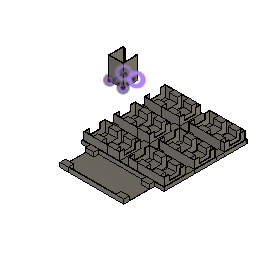
ScotlandYardInsert (Autodesk Fusion 360 design; units mm, degrees)
Autodesk Fusion 360 part; units mm, degrees
sketch "Sketch1" plane through (0, 0, 0) normal (0, 0, 1) x (1, 0, 0)
  line L0 (0, 0) -> (149.4, 0)
  line L1 (149.4, 0) -> (149.4, -151.8)
  line L2 (149.4, -151.8) -> (0, -151.8)
  line L3 (0, -151.8) -> (0, 0)
  line L4 (1.2, -1.2) -> (67.2, -1.2)
  line L5 (67.2, -1.2) -> (67.2, -41)
  line L6 (67.2, -41) -> (1.2, -41)
  line L7 (1.2, -41) -> (1.2, -1.2)
  line L8 (82.2, -1.2) -> (148.2, -1.2)
  line L9 (148.2, -41) -> (82.2, -41)
  line L10 (82.2, -41) -> (82.2, -1.2)
  line L11 (148.2, -1.2) -> (148.2, -41)
  line L12 (1.2, -56) -> (67.2, -56)
  line L13 (67.2, -95.8) -> (1.2, -95.8)
  line L14 (1.2, -95.8) -> (1.2, -56)
  line L15 (67.2, -56) -> (67.2, -95.8)
  line L16 (1.2, -110.8) -> (67.2, -110.8)
  line L17 (67.2, -150.6) -> (1.2, -150.6)
  line L18 (1.2, -150.6) -> (1.2, -110.8)
  line L19 (67.2, -110.8) -> (67.2, -150.6)
  line L20 (82.2, -56) -> (148.2, -56)
  line L21 (148.2, -95.8) -> (82.2, -95.8)
  line L22 (82.2, -95.8) -> (82.2, -56)
  line L23 (148.2, -56) -> (148.2, -95.8)
  line L24 (82.2, -110.8) -> (148.2, -110.8)
  line L25 (148.2, -150.6) -> (82.2, -150.6)
  line L26 (82.2, -150.6) -> (82.2, -110.8)
  line L27 (148.2, -110.8) -> (148.2, -150.6)
  line L28 (16.7, -151.8) -> (132.7, -151.8)
  line L29 (132.7, -151.8) -> (132.7, -208.4)
  line L30 (132.7, -208.4) -> (16.7, -208.4)
  line L31 (16.7, -208.4) -> (16.7, -151.8)
  line L32 (31.7, -153) -> (117.7, -153)
  line L33 (117.7, -153) -> (117.7, -207.2)
  line L34 (117.7, -207.2) -> (31.7, -207.2)
  line L35 (31.7, -207.2) -> (31.7, -153)
  dimension "d1" = 66
  dimension "d2" = 39.8
  dimension "d3" = 66
  dimension "d13" = 1.2
  dimension "d14" = 1.2
  dimension "d15" = 15
  dimension "d16" = 15
  dimension "d17" = 39.8
  dimension "d18" = 39.8
  dimension "d19" = 15
  dimension "d20" = 1.2
  dimension "d21" = 1.2
  dimension "d28" = 1.2
  dimension "d29" = 15
  dimension "d30" = 15
  dimension "d31" = 1.2
  dimension "d32" = 86
  dimension "d33" = 54.2
  constraint horizontal L0
  constraint vertical L1
  constraint horizontal L2
  constraint vertical L3
  constraint coincident L0.start L3.end
  constraint horizontal L4
  constraint vertical L5
  constraint horizontal L6
  constraint vertical L7
  constraint horizontal L8
  constraint vertical L11
  constraint horizontal L9
  constraint vertical L10
  constraint horizontal L12
  constraint vertical L15
  constraint horizontal L13
  constraint vertical L14
  constraint horizontal L16
  constraint vertical L19
  constraint horizontal L17
  constraint vertical L18
  constraint horizontal L20
  constraint vertical L23
  constraint horizontal L21
  constraint vertical L22
  constraint horizontal L24
  constraint vertical L27
  constraint horizontal L25
  constraint vertical L26
  constraint coincident L4.end L8
  constraint coincident L5.end L9
  constraint coincident L6.end L14
  constraint coincident L5.end L15
  constraint coincident L9.end L22
  constraint coincident L12.end L20
  constraint coincident L13.start L21
  constraint coincident L9.start L23
  constraint coincident L13.end L18
  constraint coincident L13.start L19
  constraint coincident L16.end L24
  constraint coincident L17.start L25
  constraint coincident L21.end L26
  constraint coincident L21.start L27
  constraint horizontal L28
  constraint vertical L29
  constraint horizontal L30
  constraint vertical L31
  constraint coincident L2 L28.start
  constraint horizontal L32
  constraint vertical L33
  constraint horizontal L34
  constraint vertical L35
  constraint midpoint L2 L28
  measures "d1" distance of L5 L7
  measures "d2" distance of L4 L6
  measures "d3" distance of L10 L11
  measures "d13" distance of L0 L4
  measures "d14" distance of L3 L7
  measures "d15" distance of L5 L10
  measures "d16" distance of L6 L12
  measures "d17" distance of L12 L13
  measures "d18" distance of L16 L17
  measures "d19" distance of L13 L16
  measures "d20" distance of L2 L17
  measures "d21" distance of L1 L27
  measures "d28" distance of L2 L32
  measures "d29" distance of L31 L35
  measures "d30" distance of L29 L33
  measures "d31" distance of L30 L34
  measures "d32" distance of L33 L35
  measures "d33" distance of L32 L34
extrude "Extrude1" add sketch "Sketch1" along normal blind 0.6 contours L4 L5 L6 L7 | L8 L9 L10 L11 | L12 L13 L14 L15 | L16 L17 L18 L19 | L20 L21 L22 L23 | L24 L25 L26 L27 makes body 1 at (23.2, -69.2667, 0) makes body 2 at (23.2, -14.4667, 0) makes body 3 at (45.2, -137.3333, 0) makes body 4 at (104.2, -69.2667, 0) makes body 5 at (126.2, -14.4667, 0) makes body 6 at (104.2, -124.0667, 0)
extrude "Extrude2" add sketch "Sketch1" along normal blind 6.6 contours L0 L1 L2 L3 L28 bodies 1 2 3 4 5 6
extrude "Extrude3" add sketch "Sketch1" along normal blind 0.6 separate body contours L32 L33 L34 L35 makes body 7
extrude "Extrude4" add sketch "Sketch1" along normal blind 8 contours L2 L28 L29 L30 L31 bodies 1 7
sketch "Sketch2" plane through (132.7, 0, 0) normal (1, 0, 0) x (0, 1, 0)
  line L0 (-208.4, 0) -> (-151.8, 0)
  line L1 (-151.8, 0) -> (-151.8, 6.6)
  line L2 (-151.8, 6.6) -> (-151.8, 8)
  line L3 (-151.8, 8) -> (-208.4, 8)
  line L4 (-208.4, 8) -> (-208.4, 0)
  line L5 (-198.4, 8) -> (-161.8, 8)
  line L6 (-161.8, 8) -> (-161.8, 0.6)
  line L7 (-161.8, 0.6) -> (-198.4, 0.6)
  line L8 (-198.4, 0.6) -> (-198.4, 8)
  line L9 (-151.8, 0) -> (-208.4, 0)
  dimension "d40" = 0.6
  dimension "d41" = 10
  constraint horizontal L5
  constraint vertical L6
  constraint horizontal L7
  constraint vertical L8
  constraint coincident L3 L5.start
  constraint midpoint L3 L5
  measures "d40" distance of L7 L9
  measures "d41" distance of L4 L8
extrude "Extrude5" cut sketch "Sketch2" against normal blind 116 contours L3 L5 L6 L7 L8 bodies 1
sketch "Sketch4" plane through (0, 0, 0) normal (0, 1, 0) x (-1, 0, 0)
  line L0 (-149.4, 0) -> (0, 0)
  line L1 (0, 0) -> (0, 6.6)
  line L2 (0, 6.6) -> (-149.4, 6.6)
  line L3 (-149.4, 6.6) -> (-149.4, 0)
  line L4 (-57.2, 6.6) -> (-11.2, 6.6)
  line L5 (-11.2, 6.6) -> (-11.2, 2)
  line L6 (-11.2, 2) -> (-57.2, 2)
  line L7 (-57.2, 2) -> (-57.2, 6.6)
  line L8 (-67.2, 6.6) -> (-1.2, 6.6)
  line L9 (0, 0) -> (-149.4, 0)
  line L10 (-74.7, 0) -> (-74.7, 6.6)
  line L11 (-92.2, 2) -> (-92.2, 6.6)
  line L12 (-138.2, 2) -> (-92.2, 2)
  line L13 (-92.2, 6.6) -> (-138.2, 6.6)
  line L14 (-138.2, 6.6) -> (-138.2, 2)
  dimension "d50" = 2
  dimension "d51" = 10
  constraint horizontal L4
  constraint vertical L5
  constraint horizontal L6
  constraint vertical L7
  constraint coincident L2 L4.start
  constraint midpoint L4 L8
  constraint coincident L9 L10.start
  constraint coincident L2 L10.end
  constraint perpendicular L2 L10
  constraint midpoint L2 L10.end
  constraint symmetric L4.start L10 L11.end
  constraint symmetric L4.end L10 L13.end
  constraint symmetric L5.end L10 L12.start
  constraint symmetric L6.end L10 L11.start
  measures "d50" distance of L6 L9
  measures "d51" distance of L7 L8.start
extrude "Extrude8" cut sketch "Sketch4" against normal blind 111 contours L2 L11 L12 L13 L14 | L2 L4 L5 L6 L7 L8 bodies 1
sketch "Sketch1 (2)" plane through (0, 0, 0) normal (0, 0, 1) x (1, 0, 0) in component "Krabicka"
  line L0 (66.6, -40.4) -> (1.8, -40.4)
  line L1 (1.8, -40.4) -> (1.8, -1.8)
  line L2 (1.8, -1.8) -> (66.6, -1.8)
  line L3 (66.6, -1.8) -> (66.6, -40.4)
  line L4 (65.4, -39.2) -> (59.2, -39.2)
  line L5 (59.2, -39.2) -> (59.2, -3)
  line L6 (59.2, -3) -> (65.4, -3)
  line L7 (65.4, -3) -> (65.4, -39.2)
  line L8 (44.2, -39.2) -> (33, -39.2)
  line L9 (33, -39.2) -> (33, -3)
  line L10 (33, -3) -> (44.2, -3)
  line L11 (44.2, -3) -> (44.2, -39.2)
  line L12 (18, -39.2) -> (3, -39.2)
  line L13 (3, -39.2) -> (3, -3)
  line L14 (3, -3) -> (18, -3)
  line L15 (18, -3) -> (18, -39.2)
  line L16 (67.2, -1.2) -> (67.2, -41)
  line L17 (67.2, -41) -> (57.2, -41)
  line L18 (57.2, -1.2) -> (67.2, -1.2)
  dimension "d56" = 6.2
  dimension "d57" = 1.2
  dimension "d58" = 15
  dimension "d59" = 11.2
  dimension "d60" = 15
  dimension "d61" = 15
  dimension "d62" = 1.2
  dimension "d63" = 1.2
  dimension "d74" = 1.2
  dimension "d76" = 0.6
  dimension "d77" = 0.6
  dimension "d78" = 0.6
  constraint horizontal L0
  constraint vertical L1
  constraint horizontal L2
  constraint vertical L3
  constraint horizontal L4
  constraint vertical L5
  constraint horizontal L6
  constraint vertical L7
  constraint horizontal L8
  constraint vertical L9
  constraint horizontal L10
  constraint vertical L11
  constraint horizontal L12
  constraint vertical L13
  constraint horizontal L14
  constraint vertical L15
  constraint coincident L9.end L14
  constraint coincident L5.end L10
  constraint coincident L4 L8.start
  constraint coincident L8 L12.start
  measures "d56" distance of L5 L7
  measures "d57" distance of L3 L7
  measures "d58" distance of L5 L11
  measures "d59" distance of L9 L11
  measures "d60" distance of L9 L15
  measures "d61" distance of L13 L15
  measures "d62" distance of L2 L6
  measures "d63" distance of L0 L4
  measures "d74" distance of L1 L13
  measures "d76" distance of L0 L17
  measures "d77" distance of L3 L16
  measures "d78" distance of L2 L18
extrude "Extrude1'" add sketch "Sketch1 (2)" along normal blind 0.6 separate body contours L4 L5 L6 L7 | L8 L9 L10 L11 | L12 L13 L14 L15 makes body 8 at (8, -27.1333, 0) makes body 9 at (40.4667, -27.1333, 0) makes body 10 at (61.2667, -27.1333, 0) in component "Krabicka"
extrude "Extrude2'" add sketch "Sketch1 (2)" along normal blind 20 bodies 8 9 10 in component "Krabicka"
sketch "Sketch2 (2)" plane through (66.6, 0, 0) normal (1, 0, 0) x (0, 1, 0) in component "Krabicka"
  line L0 (-40.4, 0) -> (-1.8, 0)
  line L1 (-1.8, 0) -> (-1.8, 20)
  line L2 (-1.8, 20) -> (-40.4, 20)
  line L3 (-40.4, 20) -> (-40.4, 0)
  line L4 (-31.1, 20) -> (-11.1, 20)
  line L5 (-11.1, 20) -> (-11.1, 10)
  line L6 (-11.1, 10) -> (-31.1, 10)
  line L7 (-31.1, 10) -> (-31.1, 20)
  dimension "d70" = 10
  dimension "d71" = 20
  constraint horizontal L4
  constraint vertical L5
  constraint horizontal L6
  constraint vertical L7
  constraint coincident L2 L4.start
  constraint midpoint L2 L4
  measures "d70" distance of L4 L6
  measures "d71" distance of L5 L7
extrude "Extrude3'" cut sketch "Sketch2 (2)" against normal blind 64.8 contours L2 L4 L5 L6 L7 bodies 8 in component "Krabicka"
pattern_linear "00000000-0000-0000-0000-000000000000" [suppressed]
pattern_linear "R-Pattern1" count 3 spacing 54.8 along (0, -1, 0) count 2 spacing 81 along (1, 0, 0) of bodies 8 makes body 11 at (23.4, -82.3333, 0) makes body 12 at (23.4, -137.1333, 0) makes body 13 at (104.4, -27.5333, 0) makes body 14 at (104.4, -82.3333, 0) makes body 15 at (104.4, -137.1333, 0) in component "Krabicka"
sketch "Sketch1 (3)" plane through (0, 0, 0) normal (0, 0, 1) x (1, 0, 0) in component "VytahovaciStojan"
  line L0 (-50, 0) -> (-76.8, 0)
  line L1 (-76.8, 0) -> (-76.8, -26.8)
  line L2 (-76.8, -26.8) -> (-50, -26.8)
  line L3 (-50, -26.8) -> (-50, 0)
  line L4 (-51.2, -25.6) -> (-75.6, -25.6)
  line L5 (-75.6, -25.6) -> (-75.6, -1.2)
  line L6 (-75.6, -1.2) -> (-51.2, -1.2)
  line L7 (-51.2, -1.2) -> (-51.2, -25.6)
  dimension "d87" = 26.8
  dimension "d88" = 26.8
  dimension "d90" = 1.2
  dimension "d91" = 1.2
  dimension "d93" = 1.2
  dimension "d94" = 1.2
  dimension "d96" = 50
  constraint horizontal L0
  constraint vertical L1
  constraint horizontal L2
  constraint vertical L3
  constraint horizontal L4
  constraint vertical L5
  constraint horizontal L6
  constraint vertical L7
  constraint coincident origin L0
  measures "d87" distance of L0.start L0.end
  measures "d88" distance of L0 L2
  measures "d90" distance of L3 L7
  measures "d91" distance of L0 L6
  measures "d93" distance of L2 L4
  measures "d94" distance of L1 L5
  measures "d96" distance of origin L3
extrude "Extrude1''" add sketch "Sketch1 (3)" along normal blind 0.6 separate body contours L4 L5 L6 L7 makes body 16 in component "VytahovaciStojan"
extrude "Extrude2''" add sketch "Sketch1 (3)" along normal blind 39.6 bodies 16 in component "VytahovaciStojan"
sketch "Sketch2 (3)" plane through (0, 0, 0) normal (0, 1, 0) x (-1, 0, 0) in component "VytahovaciStojan"
  line L0 (50, 0) -> (76.8, 0)
  line L1 (76.8, 0) -> (76.8, 39.6)
  line L2 (76.8, 39.6) -> (50, 39.6)
  line L3 (50, 39.6) -> (50, 0)
  line L4 (52, 1.8) -> (54, 5.8)
  line L5 (54, 11.6641) -> (54, 39.6)
  line L6 (54, 5.8) -> (54, 7)
  line L7 (54, 7) -> (52, 7)
  line L8 (52, 1.8) -> (52, 0.6)
  line L9 (52, 0.6) -> (54, 0.6)
  line L10 (54, 0.6) -> (54, 0)
  line L11 (52, 7) -> (52, 8.2)
  line L12 (52, 8.2) -> (54, 11.6641)
  line L13 (50, 0) -> (76.8, 0)
  line L14 (63.4, 0) -> (63.4, 39.6)
  line L15 (72.8, 11.6641) -> (72.8, 39.6)
  line L16 (74.8, 8.2) -> (72.8, 11.6641)
  line L17 (74.8, 7) -> (74.8, 8.2)
  line L18 (72.8, 7) -> (74.8, 7)
  line L19 (72.8, 5.8) -> (72.8, 7)
  line L20 (74.8, 1.8) -> (72.8, 5.8)
  line L21 (74.8, 1.8) -> (74.8, 0.6)
  line L22 (74.8, 0.6) -> (72.8, 0.6)
  line L23 (72.8, 0.6) -> (72.8, 0)
  dimension "d101" = 4
  dimension "d110" = 0.6
  dimension "d111" = 1.2
  dimension "d112" = 1.2
  dimension "d113" = 2
  dimension "d114" = 1.2
  dimension "d117" = 30
  dimension "d120" = 4
  dimension "d121" = 3.4641
  constraint coincident L2 L5.end
  constraint perpendicular L2 L5
  constraint vertical L6
  constraint perpendicular L6 L7
  constraint parallel L3 L8
  constraint perpendicular L8 L9
  constraint coincident L0 L10.end
  constraint perpendicular L0 L10
  constraint perpendicular L7 L11
  constraint coincident L5.start L12.end
  constraint coincident L7.end L8
  constraint midpoint L0 L14.start
  constraint midpoint L2 L14.end
  constraint coincident L4.end L10
  constraint symmetric L4.start L14 L20.start
  constraint symmetric L4.end L14 L19.start
  constraint symmetric L5.start L14 L15.start
  constraint symmetric L5.end L14 L15.end
  constraint symmetric L6.end L14 L18.start
  constraint symmetric L7.end L14 L17.start
  constraint symmetric L8.end L14 L21.end
  constraint symmetric L9.end L14 L22.end
  constraint symmetric L10.end L14 L23.end
  constraint symmetric L11.end L14 L16.start
  measures "d101" distance of L3 L5
  measures "d110" distance of L9 L13
  measures "d111" distance of L4.end L6.end
  measures "d112" distance of L4.start L8.end
  measures "d113" distance of L6.end L7.end
  measures "d114" distance of L7.end L11.end
  measures "d117" angle of L5 L12
  measures "d120" vertical distance of L4.start L4.end
  measures "d121" vertical distance of L5.start L11.end
sketch "Sketch4 (2)" plane through (0, 0, 0) normal (0, 1, 0) x (-1, 0, 0) in component "VytahovaciStojan"
  line L0 (51.2, 7) -> (75.6, 7)
  line L1 (75.6, 7) -> (75.6, 6.4)
  line L2 (75.6, 6.4) -> (51.2, 6.4)
  line L3 (51.2, 6.4) -> (51.2, 7)
  line L4 (76.8, 0) -> (76.8, 39.6)
  line L5 (50, 39.6) -> (50, 0)
  line L6 (63.4, 0) -> (63.4, 39.6)
  point P0 (72.8, 7)
  point P1 (51.2, 0)
  point P2 (75.6, 0)
  dimension "d124" = 0.6
  constraint horizontal L0
  constraint vertical L1
  constraint horizontal L2
  constraint vertical L3
  constraint coincident L0 P0
  constraint coincident L3 P1
  constraint coincident L1 P2
  measures "d124" distance of L0 L2
extrude "Extrude5'" add sketch "Sketch4 (2)" against normal blind 26 bodies 16 in component "VytahovaciStojan"
extrude "Extrude6" cut sketch "Sketch2 (3)" against normal blind 22.8 contours L0 L2 L4 L5 L6 L7 L8 L9 L10 L11 L12 L13 L14 | L0 L2 L13 L14 L15 L16 L17 L18 L19 L20 L21 L22 L23 bodies 16 in component "VytahovaciStojan"
fillet "Fillet2" radius 2 1 edges at (-72.8, -0.6, 39.6) on bodies 16 in component "VytahovaciStojan"
fillet "Fillet1" radius 2 1 edges at (-54, -0.6, 39.6) on bodies 16 in component "VytahovaciStojan"
sketch "Sketch1 (4)" plane through (0, 0, 0) normal (0, 0, 1) x (1, 0, 0) in component "Víčko"
  line L0 (-51.8, -25) -> (-75, -25)
  line L1 (-75, -25) -> (-75, -1.8)
  line L2 (-75, -1.8) -> (-51.8, -1.8)
  line L3 (-51.8, -1.8) -> (-51.8, -25)
  line L4 (-51.2, -1.2) -> (-51.2, -25.6)
  line L5 (-75.6, -25.6) -> (-75.6, -1.2)
  line L6 (-51.2, -25.6) -> (-75.6, -25.6)
  line L7 (-50, 0) -> (-52, 0)
  line L8 (-54.6, -3) -> (-72.2, -3)
  line L9 (-72.2, -3) -> (-72.2, 0)
  line L10 (-72.2, 0) -> (-54.6, 0)
  line L11 (-54.6, 0) -> (-54.6, -3)
  line L12 (-54, 0) -> (-54, -1.2)
  line L13 (-72.8, -1.2) -> (-72.8, 0)
  line L14 (-53, -3) -> (-73.8, -3)
  line L15 (-73.8, -3) -> (-73.8, -23.8)
  line L16 (-73.8, -23.8) -> (-53, -23.8)
  line L17 (-53, -23.8) -> (-53, -3)
  dimension "d139" = 0.6
  dimension "d141" = 0.6
  dimension "d142" = 0.6
  dimension "d143" = 0.6
  dimension "d144" = 0.6
  dimension "d153" = 1.2
  dimension "d154" = 1.2
  dimension "d155" = 0.6
  dimension "d156" = 1.2
  dimension "d157" = 1.2
  constraint horizontal L0
  constraint vertical L1
  constraint horizontal L2
  constraint vertical L3
  constraint horizontal L8
  constraint vertical L9
  constraint horizontal L10
  constraint vertical L11
  constraint coincident L10 L13.end
  constraint horizontal L14
  constraint vertical L15
  constraint horizontal L16
  constraint vertical L17
  constraint coincident L8.start L14
  measures "d139" distance of L3 L4
  measures "d141" distance of L0 L6
  measures "d142" distance of L2 L4.start
  measures "d143" distance of L11 L12
  measures "d144" distance of L9 L13
  measures "d153" distance of L3 L17
  measures "d154" distance of L2 L14
  measures "d155" distance of L1 L5
  measures "d156" distance of L0 L16
  measures "d157" distance of L1 L15
extrude "Extrude3''" add sketch "Sketch1 (4)" along normal blind 1.2 separate body contours L0 L1 L2 L3 L9 L11 L14 L15 L16 L17 | L8 L14 L15 L16 L17 makes body 17 in component "Víčko"
extrude "Extrude4'" add sketch "Sketch1 (4)" along normal blind 2.4 contours L2 L8 L9 L11 L14 | L2 L9 L10 L11 bodies 17 in component "Víčko"
fillet "Fillet1'" radius 1.5 2 edges at (-72.2, -1.5, 2.4) (-54.6, -1.5, 2.4) on bodies 17 in component "Víčko"
sketch "Sketch2 (4)" plane through (0, 0, 1.2) normal (0, 0, 1) x (-1, 0, 0) in component "Víčko"
  line L0 (51.8, 1.8) -> (54.6303, 1.8)
  line L1 (54.6303, 1.8) -> (54.6303, 3)
  line L2 (54.6303, 3) -> (72.1697, 3)
  line L3 (72.1697, 3) -> (72.1697, 1.8)
  line L4 (72.1697, 1.8) -> (75, 1.8)
  line L5 (75, 1.8) -> (75, 25)
  line L6 (75, 25) -> (51.8, 25)
  line L7 (51.8, 25) -> (51.8, 1.8)
  line L8 (73.8, 3) -> (73.8, 23.8)
  line L9 (53, 3) -> (73.8, 3)
  line L10 (53, 23.8) -> (53, 3)
  line L11 (73.8, 3) -> (53, 3)
  line L12 (53, 3) -> (53, 23.8)
  line L13 (53, 23.8) -> (73.8, 23.8)
  line L14 (73.8, 23.8) -> (73.8, 3)
  constraint horizontal L11
  constraint vertical L12
  constraint horizontal L13
  constraint vertical L14
  constraint coincident L10.start L12.end
  constraint coincident L8.start L9.end
extrude "Extrude5''" cut sketch "Sketch2 (4)" against normal blind 0.6 contours L2 L8 L9 L10 L11 L12 L13 L14 bodies 17 in component "Víčko"
chamfer "Chamfer1" distance 2 distance2 2.8 2 edges at (-51.2, -13.4, 6.4) (-75.6, -13.4, 6.4) measured on face at (-51.2, -9.3333, 4.4667) measured on face at (-75.6, -17.4667, 4.4667) on bodies 16 in component "VytahovaciStojan"
chamfer "Chamfer3" distance 2 distance2 2.8 1 edges at (-63.4, -25.6, 6.4) measured on face at (-66.5333, -25.6, 2.5333) on bodies 16 in component "VytahovaciStojan"
component "Krabicka" placed x (1, 0, 0) y (0, 1, 0) z (0, 0, 1) at (0, 0, 0)
component "VytahovaciStojan" placed x (1, 0, 0) y (0, 1, 0) z (0, 0, 1) at (0, 0, 0)
component "Víčko" placed x (1, 0, 0) y (0, 1, 0) z (0, 0, 1) at (0, 0, 0)
equation "d1 = 64.8 mm + 1.2 mm"
equation "d2 = 38.6 mm + 1.2 mm"
equation "d3 = 64.8 mm + 1.2 mm"
equation "d17 = 39.2 mm + 0.6 mm"
equation "d24 = 6 mm + 0.6 mm"
equation "d32 = 84.8 mm + 1.2 mm"
equation "d33 = 53 mm + 1.2 mm"
equation "d87 = 25 mm + 0.6 mm + 1.2 mm"
equation "d99 = 14.6 mm + 25 mm"
equation "d114 = ( 0.6 * 2 ) * 1 mm"
equation "d127 = -25.60 mm + 2.8 mm"
